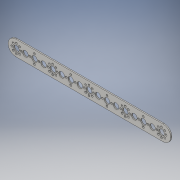
# Autodesk Inventor part: Tetrix Max Flat 288mm
Saved by Autodesk Inventor 2016 (Build 200138000, 138)
## iProperties
Created: 2015-10-23
Part Number: Tetrix Max Flat 288mm
Material: Generic
Document SubType Name: Modeling
Designer: Delta
Density: 1 g/cm^3
Appearance: Default
Author: Delta
Autodesk Inventor part; units mm, degrees
ref_plane "YZ Plane" through (0, 0, 0) normal (1, 0, 0) x (0, 1, 0)
ref_plane "XZ Plane" through (0, 0, 0) normal (0, 1, 0) x (-1, 0, 0)
ref_plane "XY Plane" through (0, 0, 0) normal (0, 0, 1) x (1, 0, 0)
sketch "Sketch1" plane through (0, 0, 0) normal (0, 0, 1) x (1, 0, 0)
  line L0 (0, 0) -> (281.7812, 0)
  line L1 (281.7812, 0) -> (281.7812, 26.57)
  line L2 (281.7812, 26.57) -> (0, 26.57)
  line L3 (0, 26.57) -> (0, 0)
  dimension "d0" = 281.7812
  dimension "d1" = 26.57
  constraints: 8 end point, 2 parallel, 1 horizontal, 1 perpendicular
  measures "d0" distance of L2.end L1.end
  measures "d1" distance of L1.end L0.end
extrude "Extrusion1" add sketch "Sketch1" along normal blind 2.04
sketch "Sketch2" plane through (0, 0, 2.04) normal (0, 0, 1) x (1, 0, 0)
  line L0 (0, 26.57) -> (0, 0) projected
  line L1 (0, 0) -> (0, 12.7584)
  line L2 (0, 12.7584) -> (14.275, 12.7584)
  line L3 (0, 12.7584) -> (14.275, 12.7584) construction
  circle A0 centre (14.275, 12.7584) radius 4.875
  line L4 (14.275, 12.7584) -> (16.815, 12.7584)
  circle A1 centre (30.005, 12.7584) radius 4.875
  circle A2 centre (45.735, 12.7584) radius 4.875
  circle A3 centre (61.465, 12.7584) radius 4.875
  circle A4 centre (77.195, 12.7584) radius 4.875
  circle A5 centre (92.925, 12.7584) radius 4.875
  circle A6 centre (108.655, 12.7584) radius 4.875
  circle A7 centre (124.385, 12.7584) radius 4.875
  circle A8 centre (140.115, 12.7584) radius 4.875
  circle A9 centre (155.845, 12.7584) radius 4.875
  circle A10 centre (171.575, 12.7584) radius 4.875
  circle A11 centre (187.305, 12.7584) radius 4.875
  circle A12 centre (203.035, 12.7584) radius 4.875
  circle A13 centre (218.765, 12.7584) radius 4.875
  circle A14 centre (234.495, 12.7584) radius 4.875
  circle A15 centre (250.225, 12.7584) radius 4.875
  circle A16 centre (265.955, 12.7584) radius 4.875
  dimension "d4" = 12.7584
  dimension "d5" = 14.275
  dimension "d6" = 0
  dimension "d7" = 9.75
  dimension "d8" = 2.54
  dimension "d13" = 15.73
  constraints: 17 centre point, 8 end point, 4 horizontal, 1 coincident, 1 collinear, 1 point on line, 48 other
  measures "d4" distance of L0.end L1.end
  measures "d5" distance of L1.end L2.end
  measures "d6" distance between parallel lines of L2 L3
  measures "d7" diameter of A0
  measures "d8" distance of L4.start L4.end
  measures "d13" distance of L4.start A1.centre
extrude "Extrusion2" cut sketch "Sketch2" against normal blind 2.04
fillet "Fillet1" radius 13.208 4 edges at (0, 26.57, 1.02) (0, 0, 1.02) (281.7812, 26.57, 1.02) (281.7812, 0, 1.02)
sketch "Sketch3" plane through (0, 0, 2.04) normal (0, 0, 1) x (1, 0, 0)
  line L0 (13.208, 0) -> (268.5733, 0) projected
  line L1 (0, 13.362) -> (0, 13.208) projected
  circle A0 centre (14.275, 12.7584) radius 4.875 projected
  line L2 (14.275, 7.8834) -> (14.275, 17.6334)
  line L3 (9.4, 12.7584) -> (19.15, 12.7584)
  line L4 (14.275, 12.7584) -> (14.275, 20.6234)
  line L5 (268.5733, 26.57) -> (13.208, 26.57) projected
  line L6 (10.8279, 9.3113) -> (17.7221, 16.2056)
  line L7 (14.275, 7.8834) -> (14.275, 17.6334)
  line L8 (17.7221, 9.3113) -> (10.8279, 16.2056)
  line L9 (19.15, 12.7584) -> (9.4, 12.7584)
  line L10 (17.7221, 16.2056) -> (10.8279, 9.3113)
  line L11 (14.275, 17.6334) -> (14.275, 7.8834)
  line L12 (10.8279, 16.2056) -> (17.7221, 9.3113)
  point P0 (0, 0)
  point P1 (8.7136, 18.3198)
  point P2 (6.41, 12.7584)
  point P3 (8.7136, 7.197)
  point P4 (14.275, 4.8934)
  point P5 (19.8364, 7.197)
  point P6 (22.14, 12.7584)
  point P7 (19.8364, 18.3198)
  dimension "d30" = 360
  dimension "d39" = 7.865
  constraints: 20 end point, 4 point on circle, 3 coincident, 1 horizontal, 1 perpendicular, 1 vertical, 39 other
  measures "d39" distance of L4.start L4.end
hole "Hole1" at (14.275, 20.6234, 2.04) at (8.7136, 18.3198, 2.04) at (6.41, 12.7584, 2.04) at (8.7136, 7.197, 2.04) at (14.275, 4.8934, 2.04) at (19.8364, 7.197, 2.04) at (22.14, 12.7584, 2.04) at (19.8364, 18.3198, 2.04) direction (0, 0, -1) diameter 3.5 end through all
pattern_linear "Rectangular Pattern1" count 5 spacing 62.92 along (1, 0, 0) of "Hole1"
sketch "Sketch4" plane through (0, 0, 2.04) normal (0, 0, 1) x (1, 0, 0)
  line L0 (45.5847, 12.7584) -> (45.5847, 20.6234)
  circle A0 centre (30.005, 12.7584) radius 4.875 projected
  line L1 (30.005, 12.7584) -> (35.5959, 12.7584)
  line L2 (30.005, 12.7584) -> (35.5959, 12.7584) construction
  line L3 (30.005, 12.7584) -> (45.5847, 12.7584)
  point P0 (0, 0)
  point P1 (37.7197, 12.7584)
  point P2 (45.5847, 4.8934)
  point P3 (53.4497, 12.7584)
  point P4 (116.3697, 12.7584)
  point P5 (108.5047, 4.8934)
  point P6 (100.6397, 12.7584)
  point P7 (108.5047, 20.6234)
  point P8 (179.2897, 12.7584)
  point P9 (171.4247, 4.8934)
  point P10 (163.5597, 12.7584)
  point P11 (171.4247, 20.6234)
  point P12 (242.2097, 12.7584)
  point P13 (234.3447, 4.8934)
  point P14 (226.4797, 12.7584)
  point P15 (234.3447, 20.6234)
  dimension "d43" = 7.865
  dimension "d46" = 360
  dimension "d48" = 0
  dimension "d49" = 15.5797
  dimension "d52" = 62.92
  constraints: 8 end point, 3 horizontal, 1 coincident, 1 collinear, 1 vertical, 17 other
  measures "d43" distance of L0.start L0.end
  measures "d48" distance between parallel lines of L1 L2
  measures "d49" distance of L1.start L0.start
  measures "d52" distance of point (53.45, 12.758) point (116.37, 12.758)
hole "Hole2" at (45.5847, 4.8934, 2.04) at (53.4497, 12.7584, 2.04) at (45.5847, 20.6234, 2.04) at (37.7197, 12.7584, 2.04) at (100.6397, 12.7584, 2.04) at (108.5047, 4.8934, 2.04) at (116.3697, 12.7584, 2.04) at (108.5047, 20.6234, 2.04) at (171.4247, 20.6234, 2.04) at (179.2897, 12.7584, 2.04) at (171.4247, 4.8934, 2.04) at (163.5597, 12.7584, 2.04) at (234.3447, 4.8934, 2.04) at (226.4797, 12.7584, 2.04) at (242.2097, 12.7584, 2.04) at (234.3447, 20.6234, 2.04) direction (0, 0, -1) diameter 3.5 end through all
body "Solid1"
